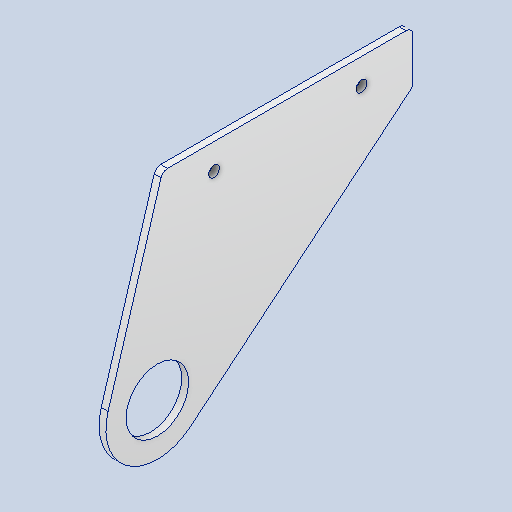
# Autodesk Inventor part: dribl-v1-Plate-1
Saved by Autodesk Inventor 2025.2 (Build 292293000, 293)
## iProperties
Created: 2025-01-04
Part Number: dribl-v1-Plate-1
Material: アルミニウム 6061
Document SubType Name: Modeling
Designer: haruy
Density: 2.7 g/cm^3
Appearance: アルミニウム - フラット
Author: haruy
Autodesk Inventor part; units mm, degrees
ref_plane "YZ Plane" through (0, 0, 0) normal (1, 0, 0) x (0, 1, 0)
ref_plane "XZ Plane" through (0, 0, 0) normal (0, 1, 0) x (-1, 0, 0)
ref_plane "XY Plane" through (0, 0, 0) normal (0, 0, 1) x (1, 0, 0)
derived "hand-grab-v3-Sketch-Base.ipt"
sketch "スケッチ1" plane through (400, 0, 0) normal (1, 0, 0) x (0, 1, 0)
  circle A0 centre (0, 0) radius 120 construction
  circle A1 centre (-96.5237, 35.1318) radius 6.5
  line L0 (0, 0) -> (-96.5237, 35.1318)
  line L1 (0, 0) -> (0, 120)
  line L2 (246.0862, 200) -> (-251.4603, 200)
  circle A2 centre (-67.6203, 200) radius 6.5
  line L3 (0, 0) -> (-120, 0)
  line L4 (248, 9.15) -> (186, 9.15)
  line L5 (186, 9.15) -> (186, -9.15)
  line L6 (186, -9.15) -> (248, -9.15)
  line L7 (248, -9.15) -> (248, 9.15)
  line L8 (186, 5.15) -> (178, 5.15)
  line L9 (178, 5.15) -> (178, -4.85)
  line L10 (178, -4.85) -> (186, -4.85)
  line L11 (186, -4.85) -> (186, 5.15)
  line L12 (178, 3.15) -> (173, 3.15)
  line L13 (173, 3.15) -> (173, -2.85)
  line L14 (173, -2.85) -> (178, -2.85)
  line L15 (178, -2.85) -> (178, 3.15)
  line L16 (173, 2.65) -> (158, 2.65)
  line L17 (158, 2.65) -> (158, -2.35)
  line L18 (158, -2.35) -> (173, -2.35)
  line L19 (173, -2.35) -> (173, 2.65)
  line L20 (186, 34.15) -> (184, 34.15)
  line L21 (184, 34.15) -> (184, -47.85)
  line L22 (184, -47.85) -> (186, -47.85)
  line L23 (186, -47.85) -> (186, 34.15)
  circle A3 centre (150, 65) radius 4
  circle A4 centre (150, 65) radius 14 construction
  line L24 (186, 34.15) -> (191, 34.15)
  line L25 (191, 34.15) -> (191, 14.15)
  line L26 (191, 14.15) -> (186, 14.15)
  line L27 (186, 14.15) -> (186, 34.15)
  line L28 (184, 34.15) -> (147.5804, 61.8148)
  line L29 (151.3835, 68.7531) -> (191, 54.15)
  line L30 (191, 54.15) -> (191, 34.15)
  line L31 (239.3868, 130) -> (-239.3868, 130)
  circle A5 centre (-96.5237, 35.1318) radius 4
  circle A6 centre (150, 65) radius 9
  line L32 (-92.7649, 33.7637) -> (-100.2825, 36.4998)
  line L33 (165, 36) -> (150, 36)
  circle A7 centre (150, 36) radius 5
  circle A8 centre (150, 36) radius 9
  circle A9 centre (-98.8174, 128.095) radius 6.5
  circle A10 centre (165, 36) radius 5
  line L34 (150, 65) -> (165, 36)
  circle A11 centre (165, 36) radius 9
  circle A12 centre (150, 65) radius 41.6497
  line L35 (150, 65) -> (150, 36)
  line L36 (150, 65) -> (-96.5237, 35.1318)
  line L37 (-98.8174, 128.095) -> (150, 65)
  line L38 (150, 65) -> (150, 23.3503)
  circle A13 centre (150, 65) radius 32.6497
  circle A14 centre (150, 32.3503) radius 9
  line L39 (166.9362, 23.3503) -> (134.8586, 23.3503)
  line L40 (174, 3.15) -> (174, -2.85)
  circle A15 centre (25, 0) radius 120
  line L41 (170, -52.2973) -> (211.3465, -67.3462)
  line L42 (211.3465, -67.3462) -> (205.1901, -84.2607)
  line L43 (205.1901, -84.2607) -> (163.8436, -69.2118)
  line L44 (163.8436, -69.2118) -> (170, -52.2973)
  line L45 (166.9218, -60.7546) -> (0, 0)
  line L46 (172.8191, -53.3234) -> (166.6627, -70.2379)
  line L47 (186, -47.85) -> (172.8191, -53.3234)
  line L48 (182.216, -56.7436) -> (176.0596, -73.6581)
  line L49 (186, -47.85) -> (191, -47.85)
  line L50 (191, -47.85) -> (191, -37.85)
  line L51 (191, -37.85) -> (186, -37.85)
  line L52 (186, -37.85) -> (186, -47.85)
  line L53 (191, -47.85) -> (182.216, -56.7436)
  circle A16 centre (221.5, -275) radius 6
  line L54 (211.5, 20) -> (208.5, 20)
  line L55 (208.5, 20) -> (208.5, -53.7075)
  line L56 (208.5, -53.7075) -> (211.5, -53.7075)
  line L57 (211.5, -53.7075) -> (211.5, 20)
  line L58 (211.5, 20) -> (231.5, 20)
  line L59 (231.5, 20) -> (231.5, -53.7075)
  line L60 (231.5, -53.7075) -> (211.5, -53.7075)
  line L61 (211.5, -53.7075) -> (211.5, 20)
  line L62 (-432.3334, -230) -> (-447.3334, -230)
  line L63 (-447.3334, -230) -> (-447.3334, -860)
  line L64 (-447.3334, -860) -> (-432.3334, -860)
  line L65 (-432.3334, -860) -> (-432.3334, -230)
  line L66 (-432.3334, -250) -> (-432.3334, -230)
  line L67 (343, -291.5) -> (278.5, -291.5)
  line L68 (278.5, -291.5) -> (278.5, -334.5)
  line L69 (278.5, -334.5) -> (343, -334.5)
  line L70 (343, -334.5) -> (343, -291.5)
  line L71 (278.5, -291.5) -> (293.5, -291.5)
  line L72 (293.5, -291.5) -> (293.5, -276.5)
  line L73 (293.5, -276.5) -> (278.5, -276.5)
  line L74 (278.5, -276.5) -> (278.5, -291.5)
  line L75 (211.5, -53.7075) -> (231.5, -53.7075)
  line L76 (231.5, -53.7075) -> (231.5, -305) construction
  line L77 (231.5, -305) -> (211.5, -305)
  line L78 (211.5, -305) -> (211.5, -53.7075) construction
  line L79 (-432.3334, -303) -> (-447.3334, -303)
  line L80 (-432.3334, -303) -> (875.6666, -303)
  line L81 (875.6666, -303) -> (875.6666, -323)
  line L82 (875.6666, -323) -> (-432.3334, -323)
  line L83 (-432.3334, -323) -> (-432.3334, -303)
  line L84 (278.5, -334.5) -> (293.5, -334.5)
  line L85 (293.5, -334.5) -> (293.5, -349.5)
  line L86 (293.5, -349.5) -> (278.5, -349.5)
  line L87 (278.5, -349.5) -> (278.5, -334.5)
  line L88 (278.5, -276.5) -> (263.5, -276.5)
  line L89 (263.5, -276.5) -> (263.5, -359.5)
  line L90 (263.5, -359.5) -> (278.5, -359.5)
  line L91 (278.5, -359.5) -> (278.5, -276.5)
  circle A17 centre (221.5, -275) radius 15
  line L92 (231.5, -275) -> (211.5, -275)
  line L93 (211.5, -275) -> (211.5, -305)
  line L94 (211.5, -305) -> (231.5, -305)
  line L95 (231.5, -305) -> (231.5, -275)
  line L96 (226.5, -266.3397) -> (216.5, -283.6603)
  line L97 (242.4808, -298.6603) -> (252.4808, -281.3397)
  line L98 (216.5, -283.6603) -> (242.4808, -298.6603)
  line L99 (-524.3334, 10.1879) -> (-524.3334, -1075.6286)
  line L100 (278.5, -349.5) -> (263.5, -349.5)
  line L101 (278.5, -276.5) -> (225.8253, -260.6372)
  line L102 (263.5, -349.5) -> (209.9279, -284.544)
  line L103 (278.5, -313) -> (263.5, -313)
  circle A18 centre (271, -291.5) radius 1.6
  circle A19 centre (271, -334.5) radius 1.6
  circle A20 centre (221.5, -275) radius 9.1
  circle A21 centre (221.5, -275) radius 50
  circle A22 centre (239.5, -334.8519) radius 12.5
  line L104 (221.5, -275) -> (237.3114, -322.4342)
  line L105 (221.5, -275) -> (178.1987, -300)
  line L106 (221.5, -275) -> (221.5, -225)
  line L107 (221.5, -275) -> (254.6735, -237.5899)
  circle A23 centre (259.5, -334.8519) radius 4
  circle A24 centre (239.5, -354.8519) radius 4
  circle A25 centre (219.5, -334.8519) radius 4
  line L108 (206.6714, -277.2613) -> (215.5457, -335.4549)
  line L109 (216.6716, -337.6803) -> (236.6716, -357.6803)
  line L110 (263.5, -349.5) -> (240.9941, -358.5624)
  circle A26 centre (259.5, -334.8519) radius 1.6
  circle A27 centre (239.5, -354.8519) radius 1.6
  circle A28 centre (219.5, -334.8519) radius 1.6
  point P0 (-60, 0)
  point P1 (875.6666, -313)
  point P2 (186, 0.15)
  point P3 (186, 0)
sketch "スケッチ2" plane through (0, 400, 0) normal (0, 1, 0) x (-1, 0, 0)
  circle A0 centre (0, 0) radius 120
  line L0 (0, 0) -> (-331.4625, 0)
  line L1 (67.5, -116.9134) -> (-135, 0)
  circle A1 centre (0, 0) radius 5
  line L2 (0, 0) -> (67.5, 116.9134)
  line L3 (0, 0) -> (67.5, -116.9134)
  line L4 (0, 0) -> (-135, 0)
  line L5 (17.0359, 37.507) -> (12.0359, 28.8468)
  line L6 (12.0359, 28.8468) -> (15.5, 26.8468)
  line L7 (15.5, 26.8468) -> (20.5, 35.507)
  line L8 (20.5, 35.507) -> (17.0359, 37.507)
  line L9 (20.5, 35.507) -> (15.5, 26.8468)
  line L10 (15.5, 26.8468) -> (18.9641, 24.8468)
  line L11 (18.9641, 24.8468) -> (23.9641, 33.507)
  line L12 (23.9641, 33.507) -> (20.5, 35.507)
  line L13 (14.5359, 33.1769) -> (21.4641, 29.1769)
  circle A2 centre (0, 0) radius 2.65
  line L14 (16.8194, 37.632) -> (10.3194, 26.3737)
  line L15 (10.3194, 26.3737) -> (5.9893, 28.8737)
  line L16 (5.9893, 28.8737) -> (12.4893, 40.132)
  line L17 (12.4893, 40.132) -> (16.8194, 37.632)
  line L18 (28.5107, 30.882) -> (24.1806, 33.382)
  line L19 (22.0107, 19.6237) -> (28.5107, 30.882)
  line L20 (24.1806, 33.382) -> (17.6806, 22.1237)
  line L21 (17.6806, 22.1237) -> (22.0107, 19.6237)
  circle A3 centre (0, 0) radius 28.3207
  line L22 (-41, 9.25) -> (-41, 4.25)
  line L23 (-41, 4.25) -> (-28, 4.25)
  line L24 (-28, 9.25) -> (-41, 9.25)
  line L25 (-28, 4.25) -> (-28, 9.25)
  line L26 (-41, -4.25) -> (-28, -4.25)
  line L27 (-41, -9.25) -> (-41, -4.25)
  line L28 (-28, -9.25) -> (-41, -9.25)
  line L29 (-28, -4.25) -> (-28, -9.25)
  line L30 (12.4893, -40.132) -> (16.8194, -37.632)
  line L31 (16.8194, -37.632) -> (10.3194, -26.3737)
  line L32 (5.9893, -28.8737) -> (12.4893, -40.132)
  line L33 (10.3194, -26.3737) -> (5.9893, -28.8737)
  line L34 (24.1806, -33.382) -> (17.6806, -22.1237)
  line L35 (28.5107, -30.882) -> (24.1806, -33.382)
  line L36 (22.0107, -19.6237) -> (28.5107, -30.882)
  line L37 (17.6806, -22.1237) -> (22.0107, -19.6237)
  line L38 (5.9893, 28.8737) -> (5.373, 27.8064)
  line L39 (22.0107, 19.6237) -> (21.3945, 18.5564)
  line L40 (-28, 9.25) -> (-26.7675, 9.25)
  line L41 (-28, -9.25) -> (-26.7675, -9.25)
  line L42 (5.9893, -28.8737) -> (2.1934, -22.2991)
  line L43 (22.0107, -19.6237) -> (21.3945, -18.5564)
  line L44 (13.6109, 31.5748) -> (3.6109, 14.2543)
  line L45 (3.6109, 14.2543) -> (-1.5853, 17.2543)
  line L46 (-1.5853, 17.2543) -> (8.4147, 34.5748)
  line L47 (8.4147, 34.5748) -> (13.6109, 31.5748)
  circle A4 centre (3.5128, 20.0844) radius 1.5
  circle A5 centre (8.5128, 28.7446) radius 1.5
  circle A6 centre (20.6372, 21.7446) radius 1.5
  circle A7 centre (15.6372, 13.0844) radius 1.5
  circle A8 centre (-29.15, 7) radius 1.5
  circle A9 centre (-19.15, 7) radius 1.5
  circle A10 centre (-19.15, -7) radius 1.5
  circle A11 centre (-29.15, -7) radius 1.5
  circle A12 centre (8.5128, -28.7446) radius 1.5
  circle A13 centre (3.5128, -20.0844) radius 1.5
  circle A14 centre (15.6372, -13.0844) radius 1.5
  circle A15 centre (20.6372, -21.7446) radius 1.5
  line L48 (1.0128, 15.7543) -> (13.6109, 31.5748)
  circle A16 centre (0, 0) radius 34.3835
  line L49 (-8, 47) -> (-188, 47)
  line L50 (-188, 47) -> (-188, 32)
  line L51 (-188, 32) -> (-8, 32)
  line L52 (-8, 32) -> (-8, 47)
ref_plane "作業平面1" through (400, 0, 0) normal (1, 0, 0) x (0, 1, 0)
ref_plane "作業平面2" through (0, 400, 0) normal (0, 1, 0) x (-1, 0, 0)
extrude "押し出し1" add sketch "スケッチ1" against normal blind 2 contours A20 L107 A17 L95 L92 | L92 L95 A17 L104 A20 | A20 L106 A17 L107 | L104 A17 L98 L96 A20 | L107 L101 A21 L88 L89 L80 L95 A17 | A17 L101 L107 | L96 L98 A17 L93 L105 A20 | L104 L98 A17 | A17 L95 L98 L104 | A20 L105 L93 L92 | L92 L93 L105 A17 L106 A20 | L98 L104 L80 L102 L93 A17 | L98 L95 L80 L104 | L93 A17 L105 | L101 L88 A21 | L93 L102 A17 | L104 L77 L102 L80 | L80 L95 L104 | L80 A21 L102 L104 L95 | L74 L68 L80 L89 A21 L88 | L104 L102 L77 | A21 L89 L80 | L80 L89 L82 A22 L102 A21 | A21 L89 L88 | L80 L68 L103 L89 | L103 L68 L82 L89 | A22 L82 L102 | A23 | L89 L102 A22 L82 | L82 L68 L87 L100 L89 | L82 A22 L102 | A26 picked at (242.6152, -322.9254) picked at (248.4191, -329.8725)
fillet "フィレット1" radius 2 3 edges at (399, 278.5, -276.5) (399, 278.5, -349.5) (399, 263.5, -349.5)
